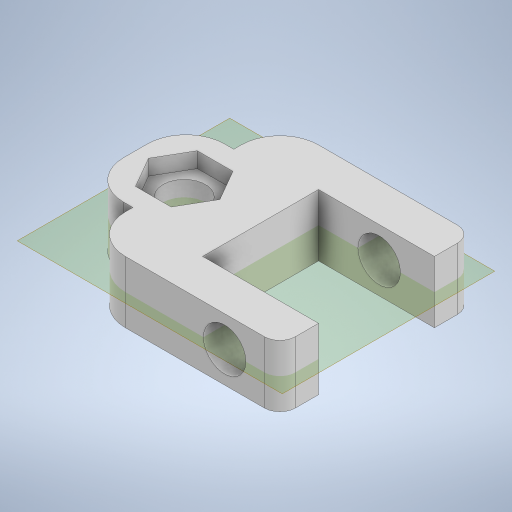
# Autodesk Inventor part: J1
Saved by Autodesk Inventor 2023 (Build 270158000, 158)
## iProperties
Created: 2023-12-18
Part Number: J1
Material: Generic
Document SubType Name: Modeling
Designer: Mustapha
Density: 1 g/cm^3
Appearance: Default
Author: Mustapha
Autodesk Inventor part; units mm, degrees
ref_plane "YZ Plane" through (0, 0, 0) normal (1, 0, 0) x (0, 1, 0)
ref_plane "XZ Plane" through (0, 0, 0) normal (0, 1, 0) x (-1, 0, 0)
ref_plane "XY Plane" through (0, 0, 0) normal (0, 0, 1) x (1, 0, 0)
sketch "Sketch1" plane through (0, 0, 0) normal (0, 1, 0) x (-1, 0, 0)
  line L0 (-10.5, 12.5) -> (7.5, 12.5)
  line L1 (12.5, 7.5) -> (12.5, -7.5)
  line L2 (7.5, -12.5) -> (-10.5, -12.5)
  line L3 (-12.5, 12.5) -> (12.5, -12.5) construction
  line L4 (12.5, 12.5) -> (-12.5, -12.5) construction
  line L5 (2.5, -7.5) -> (-12.5, -7.5)
  line L6 (-12.5, 7.5) -> (2.5, 7.5)
  line L7 (2.5, 7.5) -> (2.5, -7.5)
  line L8 (2.5, -7.5) -> (-8.1051, -8.1051) construction
  line L9 (1.2546, -1.2546) -> (2.5, 7.5) construction
  line L10 (-12.5, -10.5) -> (-12.5, -7.5)
  line L11 (-12.5, 7.5) -> (-12.5, 10.5)
  arc A0 (12.5, 7.5) -> (7.5, 12.5) centre (7.5, 7.5) ccw
  arc A1 (7.5, -12.5) -> (12.5, -7.5) centre (7.5, -7.5) ccw
  arc A2 (-10.5, 12.5) -> (-12.5, 10.5) centre (-10.5, 10.5) ccw
  arc A3 (-12.5, -10.5) -> (-10.5, -12.5) centre (-10.5, -10.5) ccw
  point P0 (0, 0)
  point P1 (-12.5, -9)
  dimension "d0" = 5
  dimension "d1" = 2
  dimension "d2" = 15
  dimension "d3" = 25
  dimension "d7" = 15
  dimension "d8" = 25
  constraints: 24 end point, 10 point on line, 8 point on circle, 8 tangent, 4 centre point, 4 parallel, 3 midpoint, 2 equal length, 2 equal radius, 2 horizontal, 1 perpendicular
  measures "d0" radius of A0
  measures "d1" radius of A2
  measures "d2" distance of L6.end L5.start
  measures "d3" distance between parallel lines of L2 L0
  measures "d7" distance of L5.start L5.end
  measures "d8" distance from line of point (-12.5, -9) L1
extrude "Extrusion1" add sketch "Sketch1" along normal blind 8
sketch "Sketch2" plane through (-7.5, 0, 12.5) normal (0, 0, 1) x (1, 0, 0)
  circle A0 centre (12.8505, 4) radius 2.75
  line L0 (0, 8) -> (18, 8) projected
  point P0 (7.5, 0)
  dimension "d9" = 5.5
  dimension "d10" = 4
  constraints: 1 centre point
  measures "d9" diameter of A0
  measures "d10" distance from line of L0 A0.centre
extrude "Extrusion2" cut sketch "Sketch2" against normal blind 44.5
sketch "Sketch4" plane through (0, 0, 0) normal (0, -1, 0) x (1, 0, 0)
  line L0 (-13.6886, 6.5298) -> (-6.3114, 6.5298)
  line L1 (-6.3114, 6.5298) -> (-6.3114, -6.5298)
  line L2 (-6.3114, -6.5298) -> (-13.6886, -6.5298)
  line L3 (-18.6886, -1.5298) -> (-18.6886, 1.5298)
  line L4 (-12.5, -7.5) -> (-12.5, 7.5) projected
  line L5 (-18.6886, 6.5298) -> (-6.3114, -6.5298) construction
  line L6 (-6.3114, 6.5298) -> (-18.6886, -6.5298) construction
  arc A0 (-18.6886, -1.5298) -> (-13.6886, -6.5298) centre (-13.6886, -1.5298) ccw
  arc A1 (-13.6886, 6.5298) -> (-18.6886, 1.5298) centre (-13.6886, 1.5298) ccw
  point P0 (0, 0)
  point P1 (-12.5, 0)
  dimension "d13" = 5
  constraints: 12 end point, 4 point on circle, 4 point on line, 4 tangent, 3 midpoint, 2 centre point, 2 parallel, 1 equal radius, 1 horizontal, 1 perpendicular
  measures "d13" radius of A0
extrude "Extrusion3" add sketch "Sketch4" against normal blind 8
sketch "Sketch5" plane through (0, 0, 0) normal (0, -1, 0) x (1, 0, 0)
  line L0 (-10.0746, -4.0008) -> (-14.6934, -4.0008)
  line L1 (-14.6934, -4.0008) -> (-17.0028, -0.0008)
  line L2 (-17.0028, -0.0008) -> (-14.6934, 3.9992)
  line L3 (-14.6934, 3.9992) -> (-10.0746, 3.9992)
  line L4 (-10.0746, 3.9992) -> (-7.7652, -0.0008)
  line L5 (-7.7652, -0.0008) -> (-10.0746, -4.0008)
  line L6 (-7.5, 12.5) -> (10.5, 12.5) projected
  circle A0 centre (-12.384, -0.0008) radius 2.75
  point P0 (0, 0)
  dimension "d16" = 8
  dimension "d17" = 5.5
  constraints: 12 end point, 1 centre point, 1 coincident, 1 parallel, 13 other
  measures "d16" distance between parallel lines of L3 L0
  measures "d17" diameter of A0
extrude "Extrusion4" cut sketch "Sketch5" against normal blind 8 contours A0
sketch "Sketch7" plane through (0, 0, 0) normal (0, -1, 0) x (1, 0, 0)
  circle A0 centre (-12.384, -0.0008) radius 2.75 projected
  line L0 (-7.7652, -0.0008) -> (-10.0746, -4.0008)
  line L1 (-10.0746, -4.0008) -> (-14.6934, -4.0008)
  line L2 (-14.6934, -4.0008) -> (-17.0028, -0.0008)
  line L3 (-17.0028, -0.0008) -> (-14.6934, 3.9992)
  line L4 (-14.6934, 3.9992) -> (-10.0746, 3.9992)
  line L5 (-10.0746, 3.9992) -> (-7.7652, -0.0008)
  line L6 (-7.5, 12.5) -> (10.5, 12.5) projected
  point P0 (0, 0)
  point P1 (-12.384, 3.9992)
  dimension "d22" = 8
  constraints: 12 end point, 1 coincident, 1 midpoint, 1 parallel, 13 other
  measures "d22" distance from line of point (-12.384, 3.999) L1
extrude "Extrusion5" cut sketch "Sketch7" against normal blind 2 contours A0 | L0 L1 L2 L3 L4 L5
ref_plane "Work Plane1" through (0, 4, 0) normal (0, -1, 0) x (1, 0, 0)
mirror "Mirror1" about plane through (0, 4, 0) normal (0, -1, 0) of "Extrusion5"
body "Solid1"
